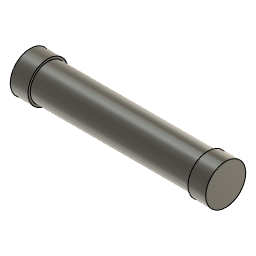
assembly v2 (Autodesk Fusion 360 archive; units mm, degrees)
design "connector"
Autodesk Fusion 360 part; units mm, degrees
sketch "Sketch1" plane through (0, 0, 0) normal (1, 0, 0) x (0, 1, 0)
  circle A0 centre (0, 0) radius 4.5
  dimension "d1" = 9
  constraint coincident A0.centre origin
  measures "d1" diameter of A0
extrude "Extrude1" add sketch "Sketch1" along normal mid plane 44
sketch "Sketch3" plane through (0, 0, 0) normal (1, 0, 0) x (0, 1, 0)
  circle A0 centre (0, 0) radius 4
  circle A1 centre (0, 0) radius 5
  dimension "d7" = 8
  dimension "d8" = 10
  constraint coincident A0.centre A1.centre
  constraint concentric A0 A1
  measures "d7" diameter of A0
  measures "d8" diameter of A1
extrude "Extrude2" cut sketch "Sketch3" along normal mid plane 36

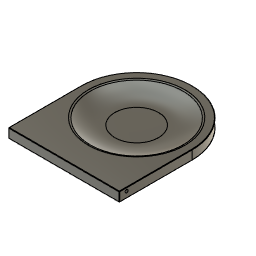
design "Base plate"
Autodesk Fusion 360 part; units mm, degrees
sketch "core" plane through (0, 0, 0) normal (0, 0, 1) x (1, 0, 0)
  circle A0 centre (0, 0) radius 152.4
  line L0 (-152.4, 0) -> (-152.4, -200)
  line L1 (-152.4, -200) -> (152.4, -200)
  line L2 (152.4, 0) -> (152.4, -200)
  dimension "d1" = 304.8
  dimension "d2" = 200
  constraint coincident A0.centre origin
  constraint coincident A0 L0.start
  constraint vertical L0
  constraint perpendicular L0 L1
  constraint coincident A0 L2.start
  constraint vertical L2
  constraint tangent A0 L2
  constraint tangent A0 L0
  measures "d1" diameter of A0
  measures "d2" distance of A0.centre L1
extrude "Extrude1" add sketch "core" along normal blind 20
sketch "plate_holder" plane through (0, 0, 0) normal (0, 1, 0) x (1, 0, 0)
  line L0 (130, -20) -> (0, -20)
  line L1 (0, -20) -> (0, -2)
  line L2 (0, -2) -> (59.9855, -2)
  arc A0 (130, -20) -> (59.9855, -2) centre (59.9855, -147.1674) ccw
  constraint horizontal L0
  constraint vertical L1
  constraint perpendicular L1 L2
  constraint tangent L2 A0
revolve "Revolve1" cut sketch "plate_holder" angle 360 about axis through (0, 0, 1.75) along (0, 0, 1)
fillet "Fillet1" radius 10 1 edges at (-121.2026, 47.01, 20)
sketch "hole1" plane through (-152.4, 0, 0) normal (-1, 0, 0) x (0, -1, 0)
  line L0 (0, 0) -> (200, 0)
  line L1 (200, 0) -> (200, 20)
  line L2 (200, 20) -> (0, 20)
  line L3 (0, 20) -> (0, 0)
  circle A0 centre (180, 10.8) radius 5
  circle A1 centre (180, 10.8) radius 4
  dimension "d8" = 10
  dimension "d9" = 20
  dimension "d10" = 9.2
  dimension "d18" = 8
  constraint concentric A0 A1
  measures "d8" diameter of A0
  measures "d9" distance of L1 A0.centre
  measures "d10" distance of L2 A0.centre
  measures "d18" diameter of A1
extrude "Extrude2" cut sketch "hole1" against normal blind 20 contours A0 | A1
extrude "Extrude4" add sketch "hole1" against normal blind 16 contours A0
sketch "hole2" plane through (152.4, 0, 0) normal (1, 0, 0) x (0, 1, 0)
  line L0 (-200, 0) -> (0, 0)
  line L1 (0, 0) -> (0, 20)
  line L2 (0, 20) -> (-200, 20)
  line L3 (-200, 20) -> (-200, 0)
  circle A0 centre (-180, 10.8) radius 5
  circle A1 centre (-180, 10.8) radius 4
  dimension "d13" = 10
  dimension "d14" = 20
  dimension "d15" = 9.2
  dimension "d21" = 8
  constraint concentric A0 A1
  measures "d13" diameter of A0
  measures "d14" distance of L3 A0.centre
  measures "d15" distance of L2 A0.centre
  measures "d21" diameter of A1
extrude "Extrude3" cut sketch "hole2" against normal blind 20 contours A0 | A1
extrude "Extrude5" add sketch "hole2" against normal blind 16 contours A0
extrude "Extrude6" add sketch "core" against normal blind 10
move_body "Move1" bodies 1 to x (1, 0, 0) y (0, 1, 0) z (0, 0, 1) at (0, 0, 10)
sketch "mirror_plane" plane through (0, -200, 0) normal (0, -1, 0) x (1, 0, 0)
  line L0 (152.4, 0) -> (152.4, 30)
  line L1 (152.4, 30) -> (-152.4, 30)
  line L2 (-152.4, 30) -> (-152.4, 0)
  line L3 (-152.4, 0) -> (152.4, 0)
  line L4 (0, 30) -> (0, 75.8638)
  line L5 (0, 75.8638, 0) -> (0, 75.8638, -67.4746)
  line L6 (-152.4, 30, -200) -> (-152.4, 30, 0)
  circle A0 through (132.5254, 30, -200) (-66.2627, 30, -85.2297) (-66.2627, 30, -314.7703)
  line L7 (0, 75.8638, -67.4746) -> (0, 30, -67.4746)
  line L8 (0, 30, -67.4746) -> (0, 30, 0)
  dimension "d27" = 90
  dimension "d29" = 90
  dimension "d30" = 152.4
  dimension "d31" = 152.4
  constraint coincident L1 L4.start
  measures "d31" distance of L1.end L4.start
extrude "Extrude8" cut sketch "core" along normal blind 4
fillet "Fillet3" radius 1 4 edges at (0, -200, 30) (152.4, -200, 17) (0, -200, 4) (-152.4, -200, 17)
fillet "Fillet4" radius 1 10 edges at (152.1071, -199.7071, 29.7071) (152.4, -99.5, 30) (0, 152.4, 30) (-152.4, -99.5, 30) (-152.1071, -199.7071, 29.7071) (152.1071, -199.7071, 4.2929) (152.4, -99.5, 4) (0, 152.4, 4) (-152.4, -99.5, 4) (-152.1071, -199.7071, 4.2929)
